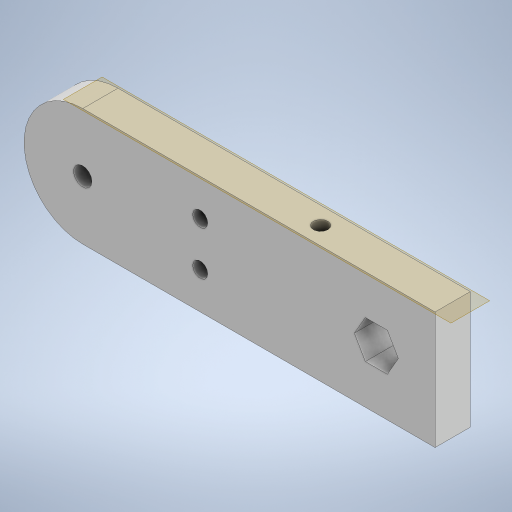
# Autodesk Inventor part: new plates for arm
Saved by Autodesk Inventor 2023 (Build 270158000, 158)
## iProperties
Created: 2023-01-16
Part Number: new plates for arm
Material: Generic
Document SubType Name: Modeling
Designer: victo
Density: 1 g/cm^3
Appearance: Default
Author: victo
Autodesk Inventor part; units mm, degrees
ref_plane "YZ Plane" through (0, 0, 0) normal (1, 0, 0) x (0, 1, 0)
ref_plane "XZ Plane" through (0, 0, 0) normal (0, 1, 0) x (-1, 0, 0)
ref_plane "XY Plane" through (0, 0, 0) normal (0, 0, 1) x (1, 0, 0)
sketch "Sketch1" plane through (0, 0, 0) normal (0, 0, 1) x (1, 0, 0)
  line L0 (-135.7759, -8.6414) -> (16.6241, -8.6414)
  line L1 (16.6241, -8.6414) -> (16.6241, -59.4414)
  line L2 (16.6241, -59.4414) -> (-135.7759, -59.4414)
  circle A0 centre (-84.9759, -24.5164) radius 3.2512
  circle A1 centre (-84.9759, -43.5664) radius 3.2512
  line L3 (-13.5384, -25.7986) -> (-4.0134, -25.7986)
  line L4 (-4.0134, -25.7986) -> (0.7491, -34.0475)
  line L5 (0.7491, -34.0475) -> (-4.0134, -42.2964)
  line L6 (-4.0134, -42.2964) -> (-13.5384, -42.2964)
  line L7 (-13.5384, -42.2964) -> (-18.3009, -34.0475)
  line L8 (-18.3009, -34.0475) -> (-13.5384, -25.7986)
  circle A2 centre (-135.7759, -34.0414) radius 3.9751
  arc A3 (-135.7759, -8.6414) -> (-135.7759, -59.4414) centre (-135.7759, -34.0414) ccw
  point P0 (0, 0)
  point P1 (-8.7759, -34.0414)
  dimension "d4" = 6.5024
  dimension "d5" = 6.5024
  dimension "d9" = 152.4
  dimension "d10" = 9.525
  dimension "d11" = 9.525
  dimension "d13" = 120
  dimension "d16" = 9.525
  dimension "d17" = 9.525
  dimension "d18" = 120
  dimension "d19" = 9.525
  dimension "d20" = 9.525
  dimension "d21" = 50.8
  dimension "d22" = 8.255
  dimension "d23" = 9.525
  dimension "d25" = 7.9502
  dimension "d27" = 9.525
  dimension "d37" = 19.05
  dimension "d38" = 50.8
  dimension "d39" = 25.4
  dimension "d40" = 50.8
  dimension "d41" = 76.2
  dimension "d42" = 25.4
  constraints: 18 end point, 4 centre point, 3 horizontal, 2 perpendicular, 2 point on circle, 1 concentric, 1 horizontal alignment, 1 point on line, 1 vertical alignment
  measures "d4" diameter of A0
  measures "d5" diameter of A1
  measures "d9" distance of L0.start L0.end
  measures "d10" distance of L3.start L3.end
  measures "d11" distance of L3.end L4.end
  measures "d13" angle of L4 L3
  measures "d16" distance of L4.end L5.end
  measures "d17" distance of L5.end L6.end
  measures "d18" angle of L5 L4
  measures "d19" distance of L6.end L7.end
  measures "d20" distance of L7.end L3.start
  measures "d21" distance of L0.end L1.end
  measures "d22" distance from line of point (-8.776, -34.041) L6
  measures "d23" distance of point (-8.776, -34.041) L7.end
  measures "d25" diameter of A2
  measures "d27" vertical distance of A2.centre A1.centre
  measures "d37" distance of A1.centre A0.centre
  measures "d38" diameter of A3
  measures "d39" distance from line of L2 A3.centre
  measures "d40" horizontal distance of A1.centre A3.centre
  measures "d41" horizontal distance of point (-8.776, -34.041) A0.centre
  measures "d42" distance from line of L1 point (-8.776, -34.041)
extrude "Extrusion1" add sketch "Sketch1" along normal blind 15.24
ref_plane "Work Plane1" through (-135.7759, -8.6414, 0) normal (0, 1, 0) x (1, 0, 0)
sketch "Sketch3" plane through (-135.7759, -8.6414, 0) normal (0, 1, 0) x (1, 0, 0)
  line L0 (50.8, -0.7344) -> (50.8, -19.7884)
  line L1 (152.4, 0) -> (152.4, -15.24) projected
  circle A0 centre (95.25, -7.62) radius 3.175
  point P0 (135.7759, 0)
  point P1 (152.4, -7.62)
  dimension "d46" = 101.6
  dimension "d47" = 6.35
  dimension "d48" = 44.45
  constraints: 2 end point, 1 centre point, 1 midpoint, 1 vertical
  measures "d46" distance from line of point (152.4, -7.62) L0
  measures "d47" diameter of A0
  measures "d48" distance from line of A0.centre L0
extrude "Extrusion2" cut sketch "Sketch3" against normal blind 50.8
body "Solid1"
